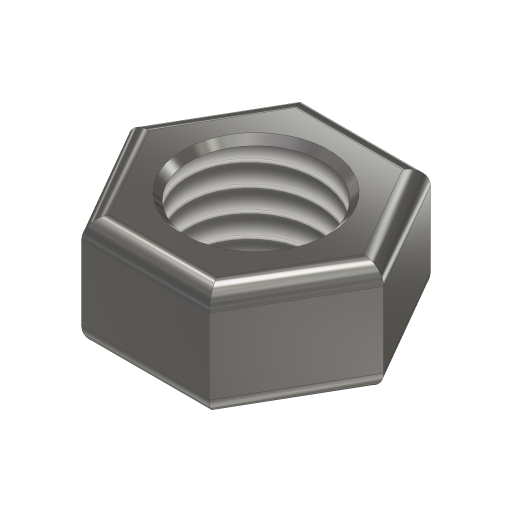
# Autodesk Inventor part: COTS_GENERIC_M6_Nut
Saved by Autodesk Inventor 2024.3 (Build 283343000, 343)
## iProperties
Created: 2018-02-17
Part Number: COTS_GENERIC_M6_Nut
Material: Ogólny
Document SubType Name: Modeling
Designer: Andrzej
Density: 1 g/cm^3
Appearance: Stal - polerowana
Mass: 0.280713 g
Surface Area: 3.53302 cm^2
Volume: 0.280713 cm^3
Author: Andrzej
Autodesk Inventor part; units mm, degrees
ref_plane "YZ Plane" through (0, 0, 0) normal (1, 0, 0) x (0, 1, 0)
ref_plane "XZ Plane" through (0, 0, 0) normal (0, 1, 0) x (-1, 0, 0)
ref_plane "XY Plane" through (0, 0, 0) normal (0, 0, 1) x (1, 0, 0)
sketch "Szkic1" plane through (0, 0, 0) normal (0, 0, 1) x (1, 0, 0)
  circle A0 centre (0, 0) radius 3
  circle A1 centre (0, 0) radius 5
  line L0 (2.8868, 5) -> (5.7735, 0)
  line L1 (5.7735, 0) -> (2.8868, -5)
  line L2 (2.8868, -5) -> (-2.8868, -5)
  line L3 (-2.8868, -5) -> (-5.7735, 0)
  line L4 (-5.7735, 0) -> (-2.8868, 5)
  line L5 (-2.8868, 5) -> (2.8868, 5)
  point P0 (0, 5)
  dimension "d1" = 10
  dimension "d0" = 6
  constraints: 12 end point, 3 coincident, 1 centre point, 1 midpoint, 1 vertical alignment, 15 other
  measures "d0" diameter of A0
extrude "Wyciągnięcie proste1" add sketch "Szkic1" along normal blind 5
fillet "Zaokrąglenie1" radius 0.8 14 edges at (1.4434, 5, 5) (-1.4434, 5, 5) (4.3301, 2.5, 5) (4.3301, -2.5, 5) (0, -5, 5) (-4.3301, -2.5, 5) (-4.3301, 2.5, 5) (1.4434, 5, 0) (-1.4434, 5, 0) (4.3301, 2.5, 0) (4.3301, -2.5, 0) (-4.3301, -2.5, 0) (-4.3301, 2.5, 0) (0, -5, 0)
chamfer "Faza1" distance 0.3 angle 45 2 edges at (-3, 0, 0) (-3, 0, 5)
thread "Gwint1" size "M6x1" class "6H" standard "ANSI Metric M Profile" full length
